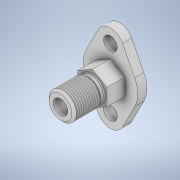
# Autodesk Inventor part: Деталь2
Saved by Autodesk Inventor 2020 (Build 240168000, 168)
## iProperties
Created: 2020-04-16
Part Number: Деталь2
Material: Типовые
Document SubType Name: Modeling
Designer: Даниил
Density: 1 g/cm^3
Appearance: По умолчанию
Mass: 50.1485 g
Surface Area: 197.878 cm^2
Volume: 50.1485 cm^3
Author: Даниил
Autodesk Inventor part; units mm, degrees
ref_plane "YZ Plane" through (0, 0, 0) normal (1, 0, 0) x (0, 1, 0)
ref_plane "XZ Plane" through (0, 0, 0) normal (0, 1, 0) x (-1, 0, 0)
ref_plane "XY Plane" through (0, 0, 0) normal (0, 0, 1) x (1, 0, 0)
sketch "Эскиз1" plane through (0, 0, 0) normal (0, 0, 1) x (1, 0, 0)
  arc A0 (-13.3609, -39.8182) -> (13.3609, -39.8182) centre (0, -33) ccw
  arc A1 (13.3609, 39.8182) -> (-13.3609, 39.8182) centre (0, 33) ccw
  line L0 (-13.3609, 39.8182) -> (-26.7217, 13.6364)
  line L1 (13.3609, 39.8182) -> (26.7217, 13.6364)
  line L2 (-26.7217, -13.6364) -> (-13.2827, -39.9713)
  line L3 (26.7217, -13.6364) -> (13.3609, -39.8182)
  arc A2 (-26.7217, 13.6364) -> (-26.7217, -13.6364) centre (0, 0) ccw
  arc A3 (26.7217, -13.6364) -> (26.7217, 13.6364) centre (0, 0) ccw
  dimension "d3" = 30
  dimension "d4" = 0
  dimension "d5" = 33
  dimension "d6" = 30
  dimension "d7" = 33
  dimension "d8" = 0
  dimension "d9" = 26.1818
  dimension "d10" = 26.1818
  constraints: 8 end point, 8 point on circle, 8 tangent, 4 centre point, 1 coincident, 1 point on line
  measures "d3" diameter of A0
  measures "d4" horizontal distance of A0.centre point (0, 0)
  measures "d5" distance of A0.centre point (0, 0)
  measures "d6" diameter of A1
  measures "d7" distance of point (0, 0) A1.centre
  measures "d8" horizontal distance of point (0, 0) A1.centre
  measures "d9" vertical distance of L0.start L0.end
  measures "d10" vertical distance of L1.start L1.end
extrude "Выдавливание1" add sketch "Эскиз1" along normal blind 10
sketch "Эскиз2" plane through (0, 0, 10) normal (0, 0, 1) x (1, 0, 0)
  circle A0 centre (0, 33) radius 7.5
  point P0 (0, 0)
  dimension "d13" = 0
  dimension "d14" = 33
  dimension "d15" = 15
  constraints: 1 centre point
  measures "d13" horizontal distance of point (0, 0) A0.centre
  measures "d14" distance of point (0, 0) A0.centre
  measures "d15" diameter of A0
extrude "Выдавливание2" cut sketch "Эскиз2" against normal blind 10
sketch "Эскиз3" plane through (0, 0, 10) normal (0, 0, 1) x (1, 0, 0)
  circle A0 centre (0, -33) radius 7.5
  point P0 (0, 0)
  dimension "d18" = 15
  dimension "d19" = 33
  dimension "d20" = 0
  constraints: 1 centre point
  measures "d18" diameter of A0
  measures "d19" distance of point (0, 0) A0.centre
  measures "d20" horizontal distance of point (0, 0) A0.centre
extrude "Выдавливание3" cut sketch "Эскиз3" against normal blind 10
sketch "Эскиз4" plane through (0, 0, 10) normal (0, 0, 1) x (1, 0, 0)
  line L0 (0, 18.5) -> (16.0215, 9.25)
  line L1 (16.0215, 9.25) -> (16.0215, -9.25)
  line L2 (16.0215, -9.25) -> (0, -18.5)
  line L3 (0, -18.5) -> (-16.0215, -9.25)
  line L4 (-16.0215, -9.25) -> (-16.0215, 9.25)
  line L5 (-16.0215, 9.25) -> (0, 18.5)
  point P0 (0, 0)
  point P1 (0, 0)
  dimension "d23" = 37
  constraints: 12 end point, 1 coincident, 1 vertical, 13 other
  measures "d23" distance of L2.end L0.start
extrude "Выдавливание4" add sketch "Эскиз4" along normal blind 20
sketch "Эскиз5" plane through (0, 0, 30) normal (0, 0, 1) x (1, 0, 0)
  circle A0 centre (0, 0) radius 13.2
  dimension "d26" = 26.4
  constraints: 1 centre point, 1 coincident
  measures "d26" diameter of A0
extrude "Выдавливание5" add sketch "Эскиз5" along normal blind 4.4
sketch "Эскиз6" plane through (0, 0, 34.4) normal (0, 0, 1) x (1, 0, 0)
  circle A0 centre (0, 0) radius 15
  dimension "d29" = 30
  constraints: 1 centre point, 1 coincident
  measures "d29" diameter of A0
extrude "Выдавливание6" add sketch "Эскиз6" along normal blind 30.6
chamfer "Фаска1" distance 2.5 angle 45 1 edges at (-15, 0, 65)
thread "Резьба1" size "M30x2.5" class "6g" standard "ANSI Metric M Profile" full length
sketch "Эскиз7" plane through (0, 0, 65) normal (0, 0, 1) x (1, 0, 0)
  circle A0 centre (0, 0) radius 8
  dimension "d37" = 16
  constraints: 1 centre point, 1 coincident
  measures "d37" diameter of A0
extrude "Выдавливание7" cut sketch "Эскиз7" against normal blind 100
sketch "Эскиз8" plane through (0, 0, 0) normal (0, 0, -1) x (-1, 0, 0)
  circle A0 centre (0, 0) radius 15
  dimension "d40" = 30
  constraints: 1 centre point, 1 coincident
  measures "d40" diameter of A0
sketch "Эскиз9" plane through (0, 0, 0) normal (1, 0, 0) x (0, 1, 0)
  point P0 (0, 0)
extrude "Выдавливание8" cut sketch "Эскиз8" against normal blind 25
fillet "Сопряжение1" radius 1.2 1 edges at (-13.2, 0, 30)
chamfer "Фаска2" distance 1.8 angle 45 1 edges at (-15, 0, 34.4)
fillet "Сопряжение3" radius 1.2 2 edges at (-13.2001, 0, 34.4) (-13.2, 0, 34.4)
chamfer "Фаска3" distance 6 angle 45 1 edges at (15, 0, 0)
sketch "Эскиз11" plane through (0, 0, 0) normal (1, 0, 0) x (0, 1, 0)
  point P0 (0, 0)
